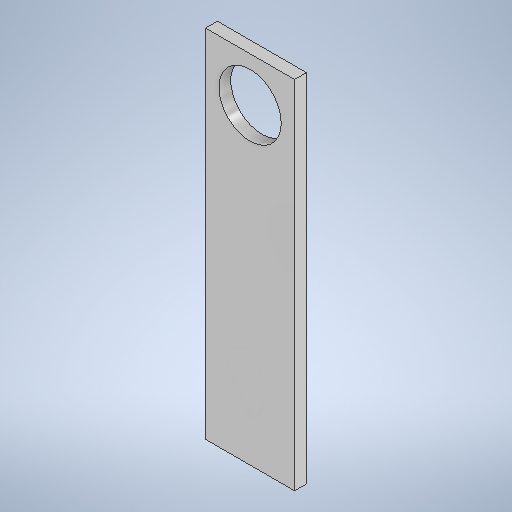
# Autodesk Inventor part: Loadcell_lever
Saved by Autodesk Inventor 2025.2 (Build 292293000, 293)
## iProperties
Created: 2026-07-22
Part Number: Loadcell_lever
Material: Generic
Document SubType Name: Modeling
Designer: Simon
Density: 1 g/cm^3
Appearance: Aluminum - Polished
Author: Simon
Autodesk Inventor part; units mm, degrees
ref_plane "YZ Plane" through (0, 0, 0) normal (1, 0, 0) x (0, 1, 0)
ref_plane "XZ Plane" through (0, 0, 0) normal (0, 1, 0) x (-1, 0, 0)
ref_plane "XY Plane" through (0, 0, 0) normal (0, 0, 1) x (1, 0, 0)
sketch "Sketch1" plane through (0, 0, 0) normal (0, 0, 1) x (1, 0, 0)
  line L0 (-7.5, -30) -> (7.5, -30)
  line L1 (7.5, -30) -> (7.5, 30)
  line L2 (7.5, 30) -> (-7.5, 30)
  line L3 (-7.5, 30) -> (-7.5, -30)
  line L4 (-7.5, -30) -> (7.5, 30) construction
  line L5 (7.5, -30) -> (-7.5, 30) construction
  line L6 (0, 30) -> (0, 22.5)
  circle A0 centre (0, 22.5) radius 5.25
  point P0 (0, 0)
  dimension "d0" = 15
  dimension "d1" = 60
  dimension "d2" = 7.5
  dimension "d3" = 10.5
  constraints: 14 end point, 3 midpoint, 2 parallel, 1 centre point, 1 coincident, 1 horizontal, 1 perpendicular, 1 vertical
  measures "d0" distance of L2.end L1.end
  measures "d1" distance of L1.end L0.end
  measures "d2" distance of L6.start L6.end
  measures "d3" diameter of A0
extrude "Extrusion1" add sketch "Sketch1" against normal blind 2
body "Solid1"
